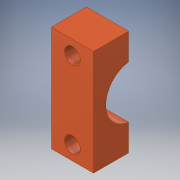
# Autodesk Inventor part: Y-axis LM8UU clamp
Saved by Autodesk Inventor 2018 (Build 220112000, 112)
## iProperties
Created: 2013-10-20
Part Number: Y-axis LM8UU clamp
Material: ABS Plastic
Document SubType Name: Modeling
Designer: Gabriel Smolnycki
Mass: 2.54516 g
Surface Area: 17.126 cm^2
Volume: 2.40109 cm^3
Density: 1.06 g/cm^3
Appearance: Smooth - Light Orange
Author: Gabriel Smolnycki
Sending System: SolidWorks 2017
Last Author: Gabriel Smolnycki
Last Saved: 2017-09-14
Autodesk Inventor part; units mm, degrees
ref_plane "XZ Plane" through (0, 0, 0) normal (0, 1, 0) x (-1, 0, 0)
ref_plane "XY Plane" through (0, 0, 0) normal (0, 0, 1) x (1, 0, 0)
ref_plane "Work Plane1" through (-6, 0, 0) normal (1, 0, 0) x (0, 1, 0)
sketch "Sketch1" plane through (-6, 0, 0) normal (1, 0, 0) x (0, 1, 0)
  line L0 (7.433, 1) -> (15, 1)
  line L1 (-15, 11) -> (-15, 1)
  arc A0 (7.433, 1) -> (-7.433, 1) centre (0, 0) ccw
  line L2 (15, 1) -> (15, 11)
  line L3 (15, 11) -> (-15, 11)
  line L4 (-15, 1) -> (-7.433, 1)
  constraints: 10 end point, 3 horizontal, 2 collinear, 2 point on circle, 2 vertical, 1 centre point
extrude "Extrusion1" add sketch "Sketch1" along normal blind 12
hole "Hole2" at (0, -11, 1) direction (0, 0, 1) diameter 4.5 depth 10 tip angle 118
sketch "Sketch2" plane through (-6, -15, 1) normal (0, 0, -1) x (-1, 0, 0)
  point P0 (-6, 4)
hole "Hole1" at (0, 11, 1) direction (0, 0, 1) diameter 4.5 depth 10 tip angle 118
sketch "Sketch3" plane through (-6, -15, 1) normal (0, 0, -1) x (-1, 0, 0)
  point P0 (-6, 26)
body "Solid3"
